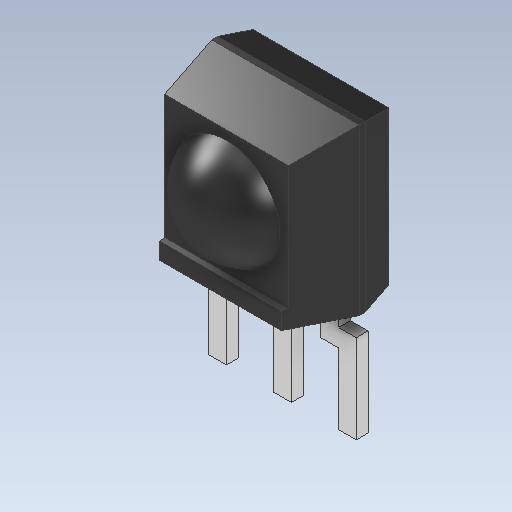
# Autodesk Inventor part: TSOP4838
Saved by Autodesk Inventor 2020 (Build 240168000, 168)
## iProperties
Created: 2020-03-25
Part Number: TSOP4838
Material: Generic
Document SubType Name: Modeling
Designer: ermoz
Density: 1 g/cm^3
Appearance: Default
Mass: 0.175504 g
Surface Area: 2.34808 cm^2
Volume: 0.175504 cm^3
Author: ermoz
Autodesk Inventor part; units mm, degrees
ref_plane "YZ Plane" through (0, 0, 0) normal (1, 0, 0) x (0, 1, 0)
ref_plane "XZ Plane" through (0, 0, 0) normal (0, 1, 0) x (-1, 0, 0)
sketch "Sketch1" plane through (0, 0, 0) normal (0, 0, 1) x (1, 0, 0)
  line L0 (-3.125, -3.125) -> (-3.125, 3.125)
  line L1 (-3.125, 3.125) -> (3.125, 3.125)
  line L2 (3.125, 3.125) -> (3.125, -3.125)
  line L3 (3.125, -3.125) -> (-3.125, 3.125) construction
  line L4 (-3.125, -3.125) -> (3.125, 3.125) construction
  line L5 (-3.125, -3.125) -> (-3.125, -3.875)
  line L6 (-3.125, -3.875) -> (3.125, -3.875)
  line L7 (3.125, -3.875) -> (3.125, -3.125)
  circle A0 centre (0, 0) radius 2.25
  line L8 (2.625, -2.625) -> (-2.625, -2.625)
  line L9 (-2.625, -2.625) -> (-2.625, 2.625)
  line L10 (-2.625, 2.625) -> (2.625, 2.625)
  line L11 (2.625, 2.625) -> (2.625, -2.625)
  line L12 (2.625, -2.625) -> (-2.625, 2.625) construction
  line L13 (-2.625, -2.625) -> (2.625, 2.625) construction
  line L14 (-3.125, -3.125) -> (-3.125, -2.625)
  line L15 (3.125, -2.625) -> (3.125, -3.125)
  line L16 (-2.625, -2.625) -> (2.625, -2.625)
  line L17 (2.625, -3.875) -> (-2.625, -3.875)
  line L18 (-2.625, -3.875) -> (2.625, -3.875)
  line L19 (2.625, -3.375) -> (-2.625, -3.375)
  line L20 (-2.625, 2.625) -> (2.625, 2.625)
  line L21 (2.625, 2.625) -> (2.625, -3.375)
  line L22 (2.625, -3.375) -> (-2.625, -3.375)
  line L23 (-2.625, -3.375) -> (-2.625, 2.625)
  line L24 (-2.625, -2.625) -> (2.625, -2.625)
  line L25 (-3.125, 3.125) -> (3.125, 3.125)
  line L26 (3.125, 3.125) -> (3.125, -3.375)
  line L27 (-3.125, -3.375) -> (-3.125, 3.125)
  line L28 (2.625, -3.375) -> (2.625, -2.625)
  line L29 (-2.625, -3.375) -> (-2.625, -2.625)
  line L30 (-2.625, -3.375) -> (-2.625, -3.875)
  line L31 (2.625, -3.375) -> (2.625, -3.875)
  line L32 (-2.625, -3.375) -> (2.625, -3.375)
  line L33 (-3.125, -3.875) -> (3.125, -3.875)
  line L34 (3.125, -3.875) -> (3.125, -2.625)
  line L35 (3.125, -2.625) -> (-3.125, -2.625)
  line L36 (-3.125, -2.625) -> (-3.125, -3.875)
  dimension "d0" = 6.25
  dimension "d1" = 6.25
  dimension "d3" = 0.75
  dimension "d4" = 4.5
  dimension "d5" = 5.25
  constraints: 74 end point, 13 parallel, 6 horizontal, 5 perpendicular, 4 midpoint, 3 point on line, 2 collinear, 2 vertical, 1 centre point, 1 coincident
  measures "d0" distance of L0.end L1.end
  measures "d1" distance of L0.start L0.end
  measures "d3" distance of L5.end L5.start
  measures "d4" diameter of A0
  measures "d5" distance of L9.end L10.end
extrude "Extrusion1" add sketch "Sketch1" against normal blind 4 contours L0 L35 L23 L30 L6 L5 | L0 L1 L2 L35 L11 L10 L9 | L9 L10 L11 L8 | L8 L21 L19 L23 | L35 L2 L7 L6 L31 L21 | L19 L31 L6 L30 | A0
extrude "Extrusion2" add sketch "Sketch1" along normal blind 0.25 contours L0 L35 L23 L30 L6 L5 | L8 L21 L19 L23 | L35 L2 L7 L6 L31 L21 | L19 L31 L6 L30
ref_plane "Work Plane1" through (-3.125, 0, 0) normal (0, 1, 0) x (1, 0, 0)
sketch "Sketch2" plane through (-3.125, 0, 0) normal (0, 1, 0) x (1, 0, 0)
  line L0 (0, -0.25) -> (0, 4) projected
  line L1 (6.25, 0) -> (0, 0) projected
  line L2 (0, 0) -> (6.25, 0)
  line L3 (3.125, 0) -> (3.125, -1.5)
  line L4 (3.125, 0) -> (5.375, 0)
  line L5 (3.125, 0) -> (0.875, 0)
  arc A0 (0.875, 0) -> (5.375, 0) centre (3.125, 0.9375) ccw
  dimension "d13" = 1.5
  dimension "d14" = 2.25
  dimension "d15" = 2.25
  constraints: 8 end point, 3 point on circle, 3 point on line, 1 centre point, 1 collinear, 1 perpendicular
  measures "d13" distance of L3.start L3.end
  measures "d14" distance of L3.start L4.end
  measures "d15" distance of L3.start L5.end
revolve "Revolution1" add sketch "Sketch2" angle 360 about axis through (0, 0, 0) along (0, 0, 1) picked at (4.5315, -0.1662) contours A0 L3 L1
chamfer "Chamfer1" distance 0.5 distance2 2.5 1 edges at (0, 3.125, 0) measured on face at (-0.0904, 2.8279, 0)
sketch "Sketch3" plane through (-3.125, -3.875, -4) normal (-1, 0, 0) x (0, 0, 1)
  line L0 (1.5, 7) -> (0, 7) projected
  line L1 (1.5, 7) -> (1.5, 0)
  line L2 (4.25, 0) -> (0, 0) projected
  line L3 (4, 0) -> (4, 0.5)
  line L4 (1.5, 0) -> (4, 0.5)
  line L5 (4, 0.5) -> (4.25, 0.55)
  line L6 (4.25, 1.25) -> (4.25, 0) projected
  line L7 (4.25, 0.55) -> (4.25, 0)
  line L8 (4.25, 0) -> (1.5, 0)
  point P0 (4, 3.875)
  dimension "d20" = 0.5
  constraints: 12 end point, 2 point on line, 2 vertical, 1 collinear, 1 perpendicular
  measures "d20" distance of L3.start L3.end
extrude "Extrusion3" cut sketch "Sketch3" against normal blind 10
sketch "Sketch4" plane through (-3.125, -3.875, -4) normal (0, -1, 0) x (1, 0, 0)
  line L0 (0, 4) -> (6.25, 4) projected
  line L1 (0, 4) -> (0.5, 4)
  line L2 (0, 1.5) -> (0, 0) projected
  line L3 (0.5, 4) -> (0, 1.5)
  line L4 (0, 4) -> (0, 4.25) projected
  line L5 (0, 1.5) -> (0, 4)
  line L6 (0, 4) -> (0, 4.25)
  line L7 (0.5, 4) -> (0.55, 4.25)
  line L8 (6.25, 4.25) -> (0, 4.25) projected
  line L9 (0.55, 4.25) -> (0, 4.25)
  line L10 (3.125, 4) -> (3.125, 3.0842)
  line L11 (6.25, 4) -> (5.75, 4)
  line L12 (5.75, 4) -> (6.25, 1.5)
  line L13 (6.25, 4) -> (6.25, 4.25)
  line L14 (6.25, 1.5) -> (6.25, 4)
  line L15 (6.25, 4) -> (6.25, 4.25)
  line L16 (5.75, 4) -> (5.7, 4.25)
  line L17 (5.7, 4.25) -> (6.25, 4.25)
  dimension "d23" = 0.5
  constraints: 28 end point, 3 symmetric about line, 2 collinear, 2 point on line, 1 horizontal, 1 vertical
  measures "d23" distance of L0.start L1.end
extrude "Extrusion4" cut sketch "Sketch4" against normal blind 10 contours L4 L8 L7 L0 | L0 L3 L5 | L16 L8 L13 L0 | L0 L14 L12
chamfer "Chamfer2" distance 1.25 distance2 0.25 1 edges at (0, 3.125, -4) measured on face at (1.0417, 3.125, -3)
chamfer "Chamfer3" distance 1.25 distance2 0.25 1 edges at (0, -3.875, -4) measured on face at (-1.0417, -3.875, -3)
chamfer "Chamfer4" distance 1.25 distance2 0.25 1 edges at (-3.125, -0.375, -4) measured on face at (-3.125, 0.7083, -3.1667)
chamfer "Chamfer5" distance 1.25 distance2 0.25 1 edges at (3.125, -0.375, -4) measured on face at (3.125, 0.7083, -3.1667)
sketch "Sketch5" plane through (-3.125, -3.875, -2.5) normal (0, -1, 0) x (1, 0, 0)
  line L0 (6.25, 0) -> (0, 0) projected
  line L1 (3.125, 0) -> (3.125, -0.25)
  line L2 (6.25, -0.25) -> (0, -0.25) projected
  line L3 (3.5, -0.375) -> (2.75, -0.375)
  line L4 (2.75, -0.375) -> (2.75, 0.125)
  line L5 (2.75, 0.125) -> (3.5, 0.125)
  line L6 (3.5, 0.125) -> (3.5, -0.375)
  line L7 (3.5, -0.375) -> (2.75, 0.125) construction
  line L8 (2.75, -0.375) -> (3.5, 0.125) construction
  point P0 (3.125, 2.5)
  point P1 (3.125, -0.125)
  dimension "d38" = 0.75
  dimension "d39" = 0.5
  constraints: 14 end point, 5 midpoint, 2 parallel, 1 horizontal, 1 perpendicular
  measures "d38" distance of L4.end L5.end
  measures "d39" distance of L3.end L4.end
extrude "Extrusion5" cut sketch "Sketch5" against normal blind 1
sketch "Sketch6" plane through (-3.125, -2.875, -2.5) normal (0, -1, 0) x (1, 0, 0)
  line L0 (2.75, -0.375) -> (2.75, 0.125) projected
  line L1 (3.5, 0.125) -> (3.5, -0.375) projected
  line L2 (2.75, 0.125) -> (3.5, 0.125)
  line L3 (3.5, 0.125) -> (3.5, -0.375)
  line L4 (3.5, -0.375) -> (2.75, -0.375)
  line L5 (2.75, -0.375) -> (2.75, 0.125)
  point P0 (3.125, 2.5)
  constraints: 8 end point, 2 parallel, 1 horizontal, 1 perpendicular
extrude "Extrusion6" add sketch "Sketch6" along normal blind 14.5 separate body
sketch "Sketch7" plane through (-3.125, -17.375, -2.5) normal (0, -1, 0) x (1, 0, 0)
  line L0 (3.5, 0.125) -> (2.75, 0.125) projected
  line L1 (2.75, -0.375) -> (3.5, -0.375) projected
  line L2 (2.75, 0.125) -> (3.5, 0.125)
  line L3 (3.5, 0.125) -> (3.5, -0.375)
  line L4 (3.5, -0.375) -> (2.75, -0.375)
  line L5 (2.75, -0.375) -> (2.75, 0.125)
  point P0 (3.125, 2.5)
  constraints: 8 end point, 2 parallel, 1 horizontal, 1 perpendicular
extrude "Extrusion7" add sketch "Sketch7" along normal blind 10 bodies 2
sketch "Sketch8" plane through (-3.125, -3.875, -2.75) normal (0, -1, 0) x (1, 0, 0)
  line L0 (2.75, 0.375) -> (3.5, 0.375) projected
  line L1 (2.75, 0.375) -> (1.5, 0.375)
  line L2 (1.5, 0.375) -> (0.75, 0.375)
  line L3 (0.75, 0.375) -> (0.75, -0.125)
  line L4 (0.75, -0.125) -> (1.5, -0.125)
  line L5 (1.5, -0.125) -> (1.5, 0.375)
  line L6 (3.5, 0.375) -> (4.75, 0.375)
  line L7 (4.75, 0.375) -> (5.5, 0.375)
  line L8 (5.5, 0.375) -> (5.5, -0.125)
  line L9 (5.5, -0.125) -> (4.75, -0.125)
  line L10 (4.75, -0.125) -> (4.75, 0.375)
  point P0 (3.125, 2.75)
  dimension "d46" = 1.25
  dimension "d47" = 0.75
  dimension "d48" = 0.5
  dimension "d49" = 1.25
  dimension "d50" = 0.75
  dimension "d51" = 0.5
  constraints: 20 end point, 4 horizontal, 4 parallel, 2 perpendicular
  measures "d46" distance of L0.start L1.end
  measures "d47" distance of L4.end L3.end
  measures "d48" distance of L3.end L2.end
  measures "d49" distance of L0.end L6.end
  measures "d50" distance of L8.end L9.end
  measures "d51" distance of L7.end L8.end
extrude "Extrusion8" cut sketch "Sketch8" against normal blind 1 bodies 1
sketch "Sketch9" plane through (-3.125, -2.875, -2.5) normal (0, 1, 0) x (1, 0, 0)
  line L0 (2.75, -0.125) -> (2.75, 0.375) projected
  line L1 (2.75, -0.125) -> (1.5, -0.125)
  line L2 (3.5, -0.125) -> (2.75, -0.125) projected
  line L3 (3.5, -0.125) -> (4.75, -0.125)
  line L4 (1.5, -0.125) -> (0.75, -0.125)
  line L5 (0.75, -0.125) -> (0.75, 0.375)
  line L6 (0.75, 0.375) -> (1.5, 0.375)
  line L7 (1.5, 0.375) -> (1.5, -0.125)
  line L8 (4.75, -0.125) -> (5.5, -0.125)
  line L9 (5.5, -0.125) -> (5.5, 0.375)
  line L10 (5.5, 0.375) -> (4.75, 0.375)
  line L11 (4.75, 0.375) -> (4.75, -0.125)
  point P0 (3.125, -2.5)
  dimension "d54" = 1.25
  dimension "d55" = 1.25
  dimension "d56" = 0.75
  dimension "d57" = 0.5
  dimension "d58" = 0.75
  dimension "d59" = 0.5
  constraints: 20 end point, 4 horizontal, 4 parallel, 2 perpendicular
  measures "d54" distance of L0.start L1.end
  measures "d55" distance of L2.start L3.end
  measures "d56" distance of L5.end L6.end
  measures "d57" distance of L4.end L5.end
  measures "d58" distance of L10.end L9.end
  measures "d59" distance of L9.end L8.end
extrude "Extrusion9" add sketch "Sketch9" against normal blind 1.75 bodies 2
sketch "Sketch10" plane through (-3.125, -4.625, -2.5) normal (0, -1, 0) x (1, 0, 0)
  line L0 (1.5, -0.375) -> (0.75, -0.375) projected
  line L1 (1.5, -0.375) -> (0, -0.375)
  line L2 (0, -0.375) -> (0, 0.125)
  line L3 (0, 0.125) -> (1.5, 0.125)
  line L4 (1.5, 0.125) -> (1.5, -0.375)
  line L5 (5.5, 0.125) -> (4.75, 0.125) projected
  line L6 (4.75, 0.125) -> (6.25, 0.125)
  line L7 (6.25, 0.125) -> (6.25, -0.375)
  line L8 (6.25, -0.375) -> (4.75, -0.375)
  line L9 (4.75, -0.375) -> (4.75, 0.125)
  point P0 (3.125, 2.5)
  dimension "d62" = 1.5
  dimension "d63" = 0.5
  dimension "d64" = 1.5
  constraints: 16 end point, 4 parallel, 2 horizontal, 2 perpendicular
  measures "d62" distance of L2.end L3.end
  measures "d63" distance of L1.end L2.end
  measures "d64" distance of L7.end L8.end
extrude "Extrusion10" add sketch "Sketch10" along normal blind 0.75 bodies 2
sketch "Sketch11" plane through (-3.125, -5.375, -2.5) normal (0, -1, 0) x (1, 0, 0)
  line L0 (0, 0.125) -> (0, -0.375) projected
  line L1 (0, -0.375) -> (0.75, -0.375) projected
  line L2 (0, 0.125) -> (0.75, 0.125)
  line L3 (0.75, 0.125) -> (0.75, -0.375)
  line L4 (0.75, -0.375) -> (0, -0.375)
  line L5 (0, -0.375) -> (0, 0.125)
  line L6 (6.25, 0.125) -> (4.75, 0.125) projected
  line L7 (5.5, -0.375) -> (6.25, -0.375) projected
  line L8 (6.25, 0.125) -> (5.5, 0.125)
  line L9 (5.5, 0.125) -> (5.5, -0.375)
  line L10 (5.5, -0.375) -> (6.25, -0.375)
  line L11 (6.25, -0.375) -> (6.25, 0.125)
  point P0 (3.125, 2.5)
  dimension "d67" = 0.75
  constraints: 16 end point, 4 parallel, 2 horizontal, 2 perpendicular
  measures "d67" distance of L1.end L4.end
extrude "Extrusion11" add sketch "Sketch11" along normal blind 22 bodies 2
sketch "Sketch12" plane through (-3.125, -27.375, -2.5) normal (0, -1, 0) x (1, 0, 0)
  line L0 (-2.9615, 1.6118) -> (7.9357, 1.6118)
  line L1 (7.9357, 1.6118) -> (7.9357, -0.9635)
  line L2 (7.9357, -0.9635) -> (-2.9615, -0.9635)
  line L3 (-2.9615, -0.9635) -> (-2.9615, 1.6118)
  point P0 (3.125, 2.5)
  constraints: 8 end point, 2 parallel, 1 horizontal, 1 perpendicular
extrude "Extrusion12" cut sketch "Sketch12" against normal blind 19 bodies 2
body "Solid1"
body "Solid2"
